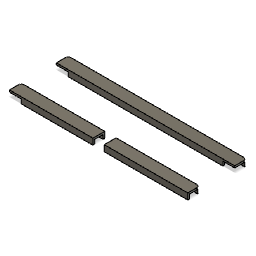
Tracks for neopixel and button v7 (Autodesk Fusion 360 design; units mm, degrees)
Autodesk Fusion 360 part; units mm, degrees
note: some values were not read from the file. Chosen so that the rebuilt part matches the saved one: which bodies a step acts on; which face or edge a step refers to.
box "BoxPrimitive1" add length 6.5 width 12.6 height 190 placed x (0, 1, 0) y (0, 0, 1) z (1, 0, 0) at (0, 0, 0.1) makes body 1
sketch "Sketch2" plane through (190, 0, 0) normal (1, 0, 0) x (0, 0, -1)
  line L0 (-0.1, 6.5) -> (-12.7, 6.5)
  line L1 (-12.7, 6.5) -> (-12.7, 0)
  line L2 (-12.7, 0) -> (-0.1, 0)
  line L3 (-0.1, 0) -> (-0.1, 6.5)
  line L4 (-6.4, 0) -> (-6.4, 2.25) construction
  line L5 (-1.9, 4.5) -> (-10.9, 4.5)
  line L6 (-10.9, 4.5) -> (-10.9, 0)
  line L7 (-10.9, 0) -> (-1.9, 0)
  line L8 (-1.9, 0) -> (-1.9, 4.5)
  line L9 (-1.9, 4.5) -> (-10.9, 0) construction
  line L10 (-10.9, 4.5) -> (-1.9, 0) construction
  point P0 (-6.4, 2.25)
  dimension "d14" = 2.25
  dimension "d15" = 9
  dimension "d16" = 4.5
  constraint midpoint L2 L4.start
  constraint perpendicular L2 L4
  constraint horizontal L5
  constraint perpendicular L5 L6
  constraint parallel L5 L7
  constraint parallel L6 L8
  constraint coincident L9 P0
  constraint coincident L10 P0
  constraint coincident P0 L4.end
  measures "d14" distance of L4.start P0
  measures "d15" distance of L6.end L7.end
  measures "d16" distance of L5.end L6.end
extrude "Extrude1" cut sketch "Sketch2" against normal blind 190 contours L2 L5 L6 L7 L8 bodies 1
copy_body "CopyPasteBodies1" bodies 1 makes body 2
move_body "Move1" bodies 2 to x (1, 0, 0) y (0, 1, 0) z (0, 0, 1) at (0, 0, -50)
sketch "Sketch3" plane through (0, 6.5, 0) normal (0, 1, 0) x (-1, 0, 0)
  line L0 (-190, 0.1) -> (0, 0.1)
  line L1 (0, 0.1) -> (0, 12.7)
  line L2 (0, 12.7) -> (-190, 12.7)
  line L3 (-190, 12.7) -> (-190, 0.1)
  line L4 (-101, 0.1) -> (-89, 0.1)
  line L5 (-89, 0.1) -> (-89, 12.7)
  line L6 (-89, 12.7) -> (-101, 12.7)
  line L7 (-101, 12.7) -> (-101, 0.1)
  line L8 (-101, 0.1) -> (-89, 12.7) construction
  line L9 (-89, 0.1) -> (-101, 12.7) construction
  line L10 (0, 6.4) -> (-95, 6.4) construction
  point P0 (-95, 6.4)
  dimension "d19" = 12
  dimension "d20" = 12.6
  dimension "d23" = 95
  constraint horizontal L4
  constraint perpendicular L4 L5
  constraint parallel L4 L6
  constraint parallel L5 L7
  constraint coincident L8 P0
  constraint coincident L9 P0
  constraint midpoint L1 L10.start
  constraint coincident P0 L10.end
  constraint perpendicular L5 L10
  measures "d19" distance of L5.end L6.end
  measures "d20" distance of L4.end L5.end
  measures "d23" distance of P0 L10.start
extrude "Extrude2" cut sketch "Sketch3" against normal blind 6.5 contours L0 L2 L4 L5 L6 L7 bodies 1 makes body 3 at (130.6667, 6.5, 8.5)
copy_body "CopyPasteBodies2" bodies 2 makes body 4
move_body "Move2" bodies 4 to x (1, 0, 0) y (0, 1, 0) z (0, 0, 1) at (0, 0, -60)
fillet "Fillet1" radius 3 4 edges at (0, 3.25, 0.1) (190, 3.25, -49.9) (0, 3.25, -49.9) (190, 3.25, 0.1) on bodies 1 2 3
sketch "Sketch6" plane through (0, 0, -37.3) normal (0, 0, 1) x (1, 0, 0)
  line L0 (190, 6.5) -> (0, 6.5)
  line L1 (0, 6.5) -> (0, 0)
  line L2 (0, 0) -> (190, 0)
  line L3 (190, 0) -> (190, 6.5)
  line L4 (12.6, 0) -> (12.6, 6.5) construction
  line L5 (177.4, 6.5) -> (177.4, 0) construction
  line L6 (190, 0) -> (177.4, 0)
  line L7 (177.4, 0) -> (177.4, 4.5)
  line L8 (177.4, 4.5) -> (190, 4.5)
  line L9 (190, 4.5) -> (190, 0)
  line L10 (0, 0) -> (12.6, 0)
  line L11 (12.6, 0) -> (12.6, 4.5)
  line L12 (12.6, 4.5) -> (0, 4.5)
  line L13 (0, 4.5) -> (0, 0)
  dimension "d27" = 12.6
  dimension "d28" = 12.6
  dimension "d29" = 12.6
  dimension "d30" = 4.5
  dimension "d31" = 12.6
  dimension "d32" = 4.5
  constraint coincident L2 L4.start
  constraint coincident L0 L4.end
  constraint perpendicular L0 L4
  constraint coincident L0 L5.start
  constraint coincident L2 L5.end
  constraint perpendicular L2 L5
  constraint horizontal L6
  constraint vertical L7
  constraint horizontal L8
  constraint vertical L9
  constraint coincident L2.end L3.start
  constraint horizontal L10
  constraint vertical L11
  constraint horizontal L12
  constraint vertical L13
  constraint coincident L1.end L2.start
  measures "d27" distance of L0.end L4.end
  measures "d28" distance of L0.start L5.start
  measures "d29" distance of L2.end L5.end
  measures "d30" distance of L2.end L8.end
  measures "d31" distance of L1.end L4.start
  measures "d32" distance of L1.end L12.end
extrude "Extrude3" cut sketch "Sketch6" against normal blind 2 contours L2 L3 L6 L7 L8 L9 | L1 L2 L10 L11 L12 L13 bodies 2
sketch "Sketch7" plane through (0, 0, 12.7) normal (0, 0, 1) x (1, 0, 0)
  line L0 (89, 0) -> (89, 6.5)
  line L1 (89, 6.5) -> (0, 6.5)
  line L2 (0, 6.5) -> (0, 0)
  line L3 (0, 0) -> (89, 0)
  line L4 (0, 0) -> (12.6, 0)
  line L5 (12.6, 0) -> (12.6, 4.5)
  line L6 (12.6, 4.5) -> (0, 4.5)
  line L7 (0, 4.5) -> (0, 0)
  dimension "d35" = 12.6
  dimension "d36" = 4.5
  constraint horizontal L4
  constraint vertical L5
  constraint horizontal L6
  constraint vertical L7
  constraint coincident L2.end L3.start
  measures "d35" distance of L2.end L4.end
  measures "d36" distance of L2.end L6.end
extrude "Extrude4" cut sketch "Sketch7" against normal blind 2 contours L2 L3 L4 L5 L6 L7 bodies 1
hidden bodies 4
equation "Length = 190 mm"
equation "Width = 12.6 mm"
equation "Depth = 6.5 mm"
equation "Lbutton = 12 mm"
equation "NeoT = 3 mm"
equation "d6 = Depth"
equation "d7 = Width"
equation "d8 = Length"
equation "Wwire = 9 mm"
equation "Hwire = 4.5 mm"
equation "d14 = Hwire / 2"
equation "d15 = Wwire"
equation "d16 = Hwire"
equation "d17 = -Length"
equation "d19 = Lbutton"
equation "d20 = Width"
equation "d21 = -Depth"
equation "d27 = Width"
equation "d28 = Width"
equation "d29 = Width"
equation "d30 = Hwire"
equation "d31 = Width"
equation "d32 = Hwire"
equation "d35 = Width"
equation "d36 = Hwire"
